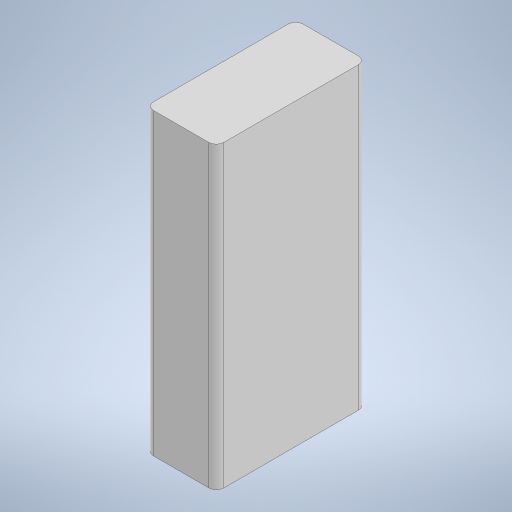
# Autodesk Inventor part: li-pol_250
Saved by Autodesk Inventor 2023 (Build 270158000, 158)
## iProperties
Created: 2024-05-17
Part Number: li-pol_250
Material: Ogólny
Document SubType Name: Modeling
Designer: kamil
Density: 1 g/cm^3
Appearance: Domyślna
Author: kamil
Autodesk Inventor part; units mm, degrees
ref_plane "YZ Plane" through (0, 0, 0) normal (1, 0, 0) x (0, 1, 0)
ref_plane "XZ Plane" through (0, 0, 0) normal (0, 1, 0) x (-1, 0, 0)
ref_plane "XY Plane" through (0, 0, 0) normal (0, 0, 1) x (1, 0, 0)
sketch "Szkic1" plane through (0, 0, 0) normal (0, 1, 0) x (-1, 0, 0)
  line L0 (2.8537, 3.2519) -> (-6.5463, 3.2519)
  line L1 (-6.5463, 3.2519) -> (-6.5463, -16.7481)
  line L2 (-6.5463, -16.7481) -> (2.8537, -16.7481)
  line L3 (2.8537, -16.7481) -> (2.8537, 3.2519)
  point P0 (0, 0)
  dimension "d0" = 9.4
  dimension "d1" = 20
  constraints: 8 end point, 2 parallel, 1 horizontal, 1 perpendicular
  measures "d0" distance of L2.end L1.end
  measures "d1" distance of L1.end L0.end
extrude "Wyciągnięcie proste1" add sketch "Szkic1" along normal blind 40
fillet "Zaokrąglenie1" radius 1 4 edges at (-2.8537, 20, -16.7481) (-2.8537, 20, 3.2519) (6.5463, 20, 3.2519) (6.5463, 20, -16.7481)
